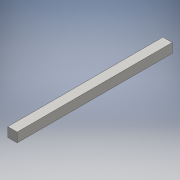
# Autodesk Inventor part: Step Motor Rod
Saved by Autodesk Inventor 2016 (Build 200138000, 138)
## iProperties
Created: 2016-05-08
Part Number: Step Motor Rod
Material: Generic
Document SubType Name: Modeling
Designer: Kenneth Daniel
Density: 1 g/cm^3
Appearance: Default
Author: Kenneth Daniel
Autodesk Inventor part; units mm, degrees
ref_plane "YZ Plane" through (0, 0, 0) normal (1, 0, 0) x (0, 1, 0)
ref_plane "XZ Plane" through (0, 0, 0) normal (0, 1, 0) x (-1, 0, 0)
ref_plane "XY Plane" through (0, 0, 0) normal (0, 0, 1) x (1, 0, 0)
sketch "Sketch1" plane through (0, 0, 0) normal (0, 1, 0) x (-1, 0, 0)
  line L0 (-1.513, 1.513) -> (-1.513, -1.513)
  line L1 (-1.513, -1.513) -> (1.513, -1.513)
  line L2 (1.513, -1.513) -> (1.513, 1.513)
  line L3 (1.513, 1.513) -> (-1.513, 1.513)
  line L4 (-1.513, 1.513) -> (1.513, -1.513) construction
  line L5 (-1.513, -1.513) -> (1.513, 1.513) construction
  point P0 (0, 0)
  dimension "d0" = 3.026
  dimension "d1" = 3.026
  constraints: 12 end point, 2 midpoint, 2 parallel, 1 perpendicular, 1 vertical
  measures "d0" distance of L0.start L0.end
  measures "d1" distance of L1.end L0.end
extrude "Extrusion1" add sketch "Sketch1" along normal blind 50
body "Solid1"
